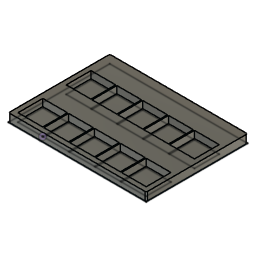
3D Printing Reference Parts (Autodesk Fusion 360 design; units mm, degrees)
Autodesk Fusion 360 part; units mm, degrees
box "BoxPrimitive1" add length 20 width 20 height 20 placed x (0, 1, 0) y (-1, 0, 0) z (0, 0, 1) at (20, 0, 0) makes body 1 in component "20x20 Cube"
sketch "Sketch1" plane through (0, 0, 0) normal (0, 0, 1) x (1, 0, 0) in component "Cube Holder"
  line L0 (0, 0) -> (-21, 0)
  line L1 (-21, 0) -> (-21, 21)
  line L2 (-21, 21) -> (0, 21)
  line L3 (0, 21) -> (0, 0)
  line L4 (22, 0) -> (1, 0)
  line L5 (1, 0) -> (1, 21)
  line L6 (1, 21) -> (22, 21)
  line L7 (22, 21) -> (22, 0)
  line L8 (44, 0) -> (23, 0)
  line L9 (23, 0) -> (23, 21)
  line L10 (23, 21) -> (44, 21)
  line L11 (44, 21) -> (44, 0)
  line L12 (66, 0) -> (45, 0)
  line L13 (45, 0) -> (45, 21)
  line L14 (45, 21) -> (66, 21)
  line L15 (66, 21) -> (66, 0)
  line L16 (88, 0) -> (67, 0)
  line L17 (67, 0) -> (67, 21)
  line L18 (67, 21) -> (88, 21)
  line L19 (88, 21) -> (88, 0)
  line L20 (0, 41) -> (-21, 41)
  line L21 (-21, 41) -> (-21, 62)
  line L22 (-21, 62) -> (0, 62)
  line L23 (0, 62) -> (0, 41)
  line L24 (22, 41) -> (1, 41)
  line L25 (1, 41) -> (1, 62)
  line L26 (1, 62) -> (22, 62)
  line L27 (22, 62) -> (22, 41)
  line L28 (44, 41) -> (23, 41)
  line L29 (23, 41) -> (23, 62)
  line L30 (23, 62) -> (44, 62)
  line L31 (44, 62) -> (44, 41)
  line L32 (66, 41) -> (45, 41)
  line L33 (45, 41) -> (45, 62)
  line L34 (45, 62) -> (66, 62)
  line L35 (66, 62) -> (66, 41)
  line L36 (88, 41) -> (67, 41)
  line L37 (67, 41) -> (67, 62)
  line L38 (67, 62) -> (88, 62)
  line L39 (88, 62) -> (88, 41)
  line L40 (92, -4) -> (-25, -4)
  line L41 (-25, -4) -> (-25, 82)
  line L42 (-25, 82) -> (92, 82)
  line L43 (92, 82) -> (92, -4)
  dimension "d8" = 21
  dimension "d9" = 21
  dimension "d12" = 22
  dimension "d13" = 41
  dimension "d14" = 4
  dimension "d15" = 4
  dimension "d16" = 20
  dimension "d17" = 20
  dimension "d18" = 4
  constraint horizontal L0
  constraint vertical L1
  constraint horizontal L2
  constraint vertical L3
  constraint coincident L0.start L3.end
  constraint horizontal L40
  constraint vertical L41
  constraint horizontal L42
  constraint vertical L43
  measures "d8" distance of L0.start L0.end
  measures "d9" distance of L0.start L2.end
  measures "d14" vertical distance of L16.start L40.start
  measures "d15" distance of L19 L43
  measures "d16" distance of L18 L36
  measures "d17" distance of L38 L42
  measures "d18" distance of L0.end L41
extrude "Extrude1" add sketch "Sketch1" along normal blind 1 separate body contours L0 L1 L2 L3 | L4 L5 L6 L7 | L8 L9 L10 L11 | L12 L13 L14 L15 | L16 L17 L18 L19 | L20 L21 L22 L23 | L24 L25 L26 L27 | L28 L29 L30 L31 | L32 L33 L34 L35 | L36 L37 L38 L39 makes body 2 at (30, 48, 0) makes body 3 at (52, 7, 0) makes body 4 at (-7, 7, 0) makes body 5 at (74, 7, 0) makes body 6 at (15, 48, 0) makes body 7 at (52, 48, 0) makes body 8 at (37, 14, 0) makes body 9 at (8, 7, 0) makes body 10 at (74, 48, 0) makes body 11 at (-7, 48, 0) in component "Cube Holder"
extrude "Extrude2" add sketch "Sketch1" along normal blind 7 bodies 2 3 4 5 6 7 8 9 10 11 in component "Cube Holder"
fillet "Fillet1" radius 1 4 edges at (92, -4, 3.5) (-25, -4, 3.5) (-25, 82, 3.5) (92, 82, 3.5) on bodies 2 in component "Cube Holder"
component "20x20 Cube" placed x (1, 0, 0) y (0, 1, 0) z (0, 0, 1) at (0, 0, 0)
component "Cube Holder" placed x (1, 0, 0) y (0, 1, 0) z (0, 0, 1) at (0, 0, 0)
equation "d14 = d15"
equation "d17 = d16"
equation "d18 = d15"
named bodies: "Base"
